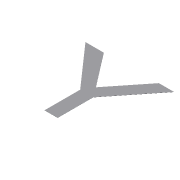
# Autodesk Inventor part: Y
Saved by Autodesk Inventor 2014 (Build 180170000, 170)
## iProperties
Created: 2014-02-18
Part Number: Y
Material: Generic
Document SubType Name: Modeling
Designer: Yogesh
Density: 1 g/cm^3
Appearance: Default
Author: Yogesh
Autodesk Inventor part; units mm, degrees
ref_plane "YZ Plane" through (0, 0, 0) normal (1, 0, 0) x (0, 1, 0)
ref_plane "XZ Plane" through (0, 0, 0) normal (0, 1, 0) x (-1, 0, 0)
ref_plane "XY Plane" through (0, 0, 0) normal (0, 0, 1) x (1, 0, 0)
sketch "Sketch1" plane through (0, 0, 0) normal (0, 0, 1) x (1, 0, 0)
  line L0 (1756.3375, 7257.8135) -> (3194.8729, 7257.8135)
  line L1 (3194.8729, 7257.8135) -> (5230.9819, 4602.0192)
  line L2 (5230.9819, 4602.0192) -> (7413.236, 7346.0417)
  line L3 (7413.236, 7346.0417) -> (8601.5922, 7346.0417)
  line L4 (8601.5922, 7346.0417) -> (5799.5547, 3822.6876)
  line L5 (5799.5547, 3822.6876) -> (5799.5547, 1036.9506)
  line L6 (5799.5547, 1036.9506) -> (4777.2459, 1036.9506)
  line L7 (4777.2459, 1036.9506) -> (4777.2459, 3822.6876)
  line L8 (4777.2459, 3822.6876) -> (1756.3375, 7257.8135)
  point P0 (0, 0)
  constraints: 18 end point, 3 parallel, 2 perpendicular, 1 horizontal
extrude "Extrusion1" add sketch "Sketch1" along normal blind 10
body "Solid1"
